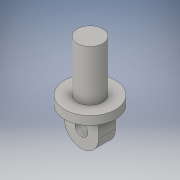
# Autodesk Inventor part: shock absorber bottom
Saved by Autodesk Inventor 2016 (Build 200138000, 138)
## iProperties
Created: 2017-06-27
Part Number: shock absorber bottom
Material: Generic
Document SubType Name: Modeling
Designer: andon
Density: 1 g/cm^3
Appearance: Default
Author: andon
Autodesk Inventor part; units mm, degrees
ref_plane "YZ Plane" through (0, 0, 0) normal (1, 0, 0) x (0, 1, 0)
ref_plane "XZ Plane" through (0, 0, 0) normal (0, 1, 0) x (-1, 0, 0)
ref_plane "XY Plane" through (0, 0, 0) normal (0, 0, 1) x (1, 0, 0)
sketch "Sketch1" plane through (0, 0, 0) normal (0, 0, 1) x (1, 0, 0)
  line L0 (-19.05, 38.1) -> (0, 38.1)
  line L1 (-19.05, -38.1) -> (-19.05, 38.1)
  line L2 (-38.1, -50.8) -> (-38.1, -38.1)
  line L3 (-19.05, -38.1) -> (-38.1, -38.1)
  line L4 (-38.1, -50.8) -> (0, -50.8)
  line L5 (0, 38.1) -> (0, -50.8)
  line L6 (0, -68.58) -> (0, 55.88) projected
  point P0 (0, 0)
  constraints: 12 end point, 1 horizontal
revolve "Revolution1" add sketch "Sketch1" angle 360 about axis through (0, -10, 0) along (0, 1, 0)
sketch "Sketch2" plane through (0, -50.8, 0) normal (0, -1, 0) x (1, 0, 0)
  line L0 (25.4, 25.4) -> (-25.4, 25.4)
  line L1 (-25.4, 25.4) -> (-25.4, -25.4)
  line L2 (-25.4, -25.4) -> (25.4, -25.4)
  line L3 (25.4, -25.4) -> (25.4, 25.4)
  line L4 (25.4, 25.4) -> (-25.4, -25.4) construction
  line L5 (-25.4, 25.4) -> (25.4, -25.4) construction
  line L6 (25.4, 12.7) -> (-25.4, 12.7)
  line L7 (-25.4, 12.7) -> (-25.4, -12.7)
  line L8 (-25.4, -12.7) -> (25.4, -12.7)
  line L9 (25.4, -12.7) -> (25.4, 12.7)
  point P0 (0, 0)
  dimension "d5" = 50.8
  dimension "d6" = 50.8
  constraints: 20 end point, 4 parallel, 2 horizontal, 2 midpoint, 2 perpendicular, 2 point on line
  measures "d5" distance of L2.end L1.end
  measures "d6" distance of L1.end L0.end
extrude "Extrusion3" add sketch "Sketch2" along normal blind 50.8 contours L3 L8 L1 L6
fillet "Fillet2" radius 25.4 2 edges at (25.4, -101.6, 0) (-25.4, -101.6, 0)
sketch "Sketch4" plane through (-25.4, -50.8, 12.7) normal (0, 0, 1) x (1, 0, 0)
  arc A0 (0, -25.4) -> (50.8, -25.4) centre (25.4, -25.4) ccw projected
  line L0 (50.8, 0) -> (50.8, -25.4) projected
  line L1 (0, 0) -> (50.8, 0) projected
  line L2 (0, 0) -> (0, -25.4) projected
  circle A1 centre (25.4, -25.4) radius 9.525
  point P0 (25.4, 50.8)
  dimension "d16" = 19.05
  constraints: 1 centre point, 1 coincident
  measures "d16" diameter of A1
extrude "Extrusion4" cut sketch "Sketch4" against normal blind 50.8 contours A1
body "Solid1"
